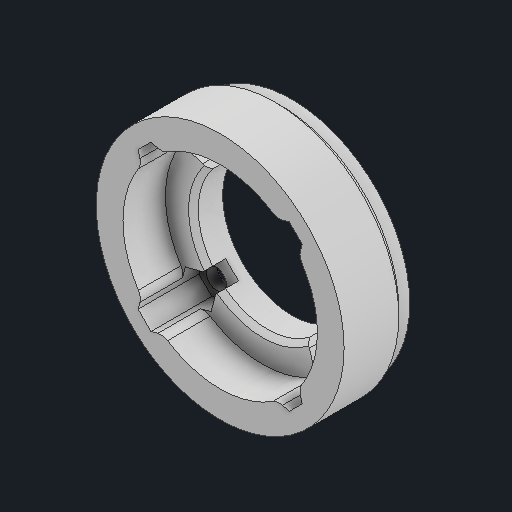
# Autodesk Inventor part: ShaftLock_A
Saved by Autodesk Inventor 2025.1 (Build 291241020, 241B)
## iProperties
Created: 2025-07-24
Part Number: ShaftLock_A
Material: 일반
Document SubType Name: Modeling
Designer: acalo
Density: 1 g/cm^3
Appearance: 기본값
Author: acalo
Autodesk Inventor part; units mm, degrees
ref_plane "YZ Plane" through (0, 0, 0) normal (1, 0, 0) x (0, 1, 0)
ref_plane "XZ Plane" through (0, 0, 0) normal (0, 1, 0) x (-1, 0, 0)
ref_plane "XY Plane" through (0, 0, 0) normal (0, 0, 1) x (1, 0, 0)
sketch "스케치1" plane through (0, 0, 0) normal (0, 0, 1) x (1, 0, 0)
  circle A0 centre (0, 0) radius 19.4
  circle A1 centre (10.6066, 10.6066) radius 1.65
  circle A2 centre (0, 0) radius 11
  circle A3 centre (-10.6066, 10.6066) radius 1.65
  circle A4 centre (-10.6066, -10.6066) radius 1.65
  circle A5 centre (10.6066, -10.6066) radius 1.65
  dimension "d1" = 22
  dimension "d5" = 360
  constraints: 6 centre point, 1 coincident, 9 other
  measures "d1" diameter of A2
extrude "돌출1" add sketch "스케치1" along normal blind 4.8
sketch "스케치2" plane through (0, 0, 4.8) normal (0, 0, 1) x (1, 0, 0)
  circle A0 centre (0, 0) radius 19.4 projected
  circle A1 centre (10.6066, -10.6066) radius 1.65 projected
  circle A2 centre (-10.6066, -10.6066) radius 1.65 projected
  circle A3 centre (-10.6066, 10.6066) radius 1.65 projected
  circle A4 centre (0, 0) radius 11 projected
  circle A5 centre (10.6066, 10.6066) radius 1.65 projected
  line L0 (10.6066, 10.6066) -> (8.8388, 8.8388)
  line L1 (10.6066, 10.6066) -> (13.1066, 10.6066) construction
  line L2 (7.8182, 9.8595) -> (8.5654, 12.6478)
  line L3 (8.5654, 12.6478) -> (11.3537, 13.395)
  line L4 (11.3537, 13.395) -> (13.395, 11.3537)
  line L5 (13.395, 11.3537) -> (12.6478, 8.5654)
  line L6 (12.6478, 8.5654) -> (9.8595, 7.8182)
  line L7 (9.8595, 7.8182) -> (7.8182, 9.8595)
  line L8 (-10.6066, 10.6066) -> (-10.6066, 13.1066) construction
  line L9 (-13.395, 11.3537) -> (-11.3537, 13.395)
  line L10 (-11.3537, 13.395) -> (-8.5654, 12.6478)
  line L11 (-8.5654, 12.6478) -> (-7.8182, 9.8595)
  line L12 (-7.8182, 9.8595) -> (-9.8595, 7.8182)
  line L13 (-12.6478, 8.5654) -> (-13.395, 11.3537)
  line L14 (-9.8595, 7.8182) -> (-12.6478, 8.5654)
  line L15 (-10.6066, -10.6066) -> (-13.1066, -10.6066) construction
  line L16 (-11.3537, -13.395) -> (-13.395, -11.3537)
  line L17 (-13.395, -11.3537) -> (-12.6478, -8.5654)
  line L18 (-12.6478, -8.5654) -> (-9.8595, -7.8182)
  line L19 (-9.8595, -7.8182) -> (-7.8182, -9.8595)
  line L20 (-8.5654, -12.6478) -> (-11.3537, -13.395)
  line L21 (-7.8182, -9.8595) -> (-8.5654, -12.6478)
  line L22 (10.6066, -10.6066) -> (10.6066, -13.1066) construction
  line L23 (13.395, -11.3537) -> (11.3537, -13.395)
  line L24 (11.3537, -13.395) -> (8.5654, -12.6478)
  line L25 (8.5654, -12.6478) -> (7.8182, -9.8595)
  line L26 (7.8182, -9.8595) -> (9.8595, -7.8182)
  line L27 (12.6478, -8.5654) -> (13.395, -11.3537)
  line L28 (9.8595, -7.8182) -> (12.6478, -8.5654)
  point P0 (-8.8388, 8.8388)
  point P1 (-8.8388, -8.8388)
  point P2 (8.8388, -8.8388)
  dimension "d9" = 2.5
  dimension "d10" = 135
  dimension "d13" = 360
  constraints: 58 end point, 1 coincident, 1 equal length, 1 horizontal, 1 midpoint, 78 other
  measures "d9" distance of L0.start L0.end
  measures "d10" angle of L0 L1
extrude "돌출2" cut sketch "스케치2" against normal blind 3 contours A1 | A2 | A3 | A5 | L7 L2 L3 L4 L5 L6 | L9 L10 L11 L12 L14 L13 | L16 L17 L18 L19 L21 L20 | L23 L24 L25 L26 L28 L27
sketch "스케치3" plane through (0, 0, 4.8) normal (0, 0, 1) x (1, 0, 0)
  circle A0 centre (0, 0) radius 16
  circle A1 centre (0, 0) radius 22.4
  line L0 (-7.8182, 9.8595) -> (-9.8595, 7.8182) projected
  line L1 (-9.8595, 7.8182) -> (-12.6478, 8.5654) projected
  line L2 (-12.6478, 8.5654) -> (-13.395, 11.3537) projected
  line L3 (-13.395, 11.3537) -> (-11.3537, 13.395) projected
  line L4 (-11.3537, 13.395) -> (-8.5654, 12.6478) projected
  line L5 (-8.5654, 12.6478) -> (-7.8182, 9.8595) projected
  line L6 (-9.8595, -7.8182) -> (-7.8182, -9.8595) projected
  line L7 (-7.8182, -9.8595) -> (-8.5654, -12.6478) projected
  line L8 (-8.5654, -12.6478) -> (-11.3537, -13.395) projected
  line L9 (-11.3537, -13.395) -> (-13.395, -11.3537) projected
  line L10 (-13.395, -11.3537) -> (-12.6478, -8.5654) projected
  line L11 (-12.6478, -8.5654) -> (-9.8595, -7.8182) projected
  line L12 (13.395, 11.3537) -> (12.6478, 8.5654) projected
  line L13 (12.6478, 8.5654) -> (9.8595, 7.8182) projected
  line L14 (9.8595, 7.8182) -> (7.8182, 9.8595) projected
  line L15 (7.8182, 9.8595) -> (8.5654, 12.6478) projected
  line L16 (8.5654, 12.6478) -> (11.3537, 13.395) projected
  line L17 (11.3537, 13.395) -> (13.395, 11.3537) projected
  line L18 (7.8182, -9.8595) -> (9.8595, -7.8182) projected
  line L19 (9.8595, -7.8182) -> (12.6478, -8.5654) projected
  line L20 (12.6478, -8.5654) -> (13.395, -11.3537) projected
  line L21 (13.395, -11.3537) -> (11.3537, -13.395) projected
  line L22 (11.3537, -13.395) -> (8.5654, -12.6478) projected
  line L23 (8.5654, -12.6478) -> (7.8182, -9.8595) projected
  circle A2 centre (0, 0) radius 19.4 projected
  circle A3 centre (0, 0) radius 11 projected
  point P0 (-9.4762, 12.8919)
  point P1 (9.4762, 12.8919)
  point P2 (12.8919, 9.4762)
  point P3 (12.8919, -9.4762)
  point P4 (9.4762, -12.8919)
  point P5 (-9.4762, -12.8919)
  point P6 (-12.8919, -9.4762)
  point P7 (-12.8919, 9.4762)
  dimension "d17" = 32
  dimension "d18" = 6.4
  constraints: 2 centre point, 1 coincident
  measures "d17" diameter of A0
  measures "d18" radial gap between concentric circles of A0 A1
extrude "돌출3" add sketch "스케치3" along normal blind 7 contours A1 | A2
chamfer "모따기1" distance 3 angle 45 1 edges at (-19.4, 0, 4.8)
sketch "스케치4" plane through (0, 0, 4.8) normal (0, 0, 1) x (1, 0, 0)
  circle A0 centre (0, 0) radius 11 projected
  arc A1 (12.8919, -9.4762) -> (12.8919, 9.4762) centre (0, 0) ccw projected
  line L0 (12.8919, 9.4762) -> (12.6478, 8.5654) projected
  line L1 (12.6478, 8.5654) -> (9.8595, 7.8182) projected
  line L2 (9.8595, 7.8182) -> (7.8182, 9.8595) projected
  line L3 (7.8182, 9.8595) -> (8.5654, 12.6478) projected
  line L4 (8.5654, 12.6478) -> (9.4762, 12.8919) projected
  arc A2 (9.4762, 12.8919) -> (-9.4762, 12.8919) centre (0, 0) ccw projected
  line L5 (-9.4762, 12.8919) -> (-8.5654, 12.6478) projected
  line L6 (-8.5654, 12.6478) -> (-7.8182, 9.8595) projected
  line L7 (-7.8182, 9.8595) -> (-9.8595, 7.8182) projected
  line L8 (-9.8595, 7.8182) -> (-12.6478, 8.5654) projected
  line L9 (-12.6478, 8.5654) -> (-12.8919, 9.4762) projected
  arc A3 (-12.8919, 9.4762) -> (-12.8919, -9.4762) centre (0, 0) ccw projected
  line L10 (-12.8919, -9.4762) -> (-12.6478, -8.5654) projected
  line L11 (-12.6478, -8.5654) -> (-9.8595, -7.8182) projected
  line L12 (-9.8595, -7.8182) -> (-7.8182, -9.8595) projected
  line L13 (-7.8182, -9.8595) -> (-8.5654, -12.6478) projected
  line L14 (-8.5654, -12.6478) -> (-9.4762, -12.8919) projected
  arc A4 (-9.4762, -12.8919) -> (9.4762, -12.8919) centre (0, 0) ccw projected
  line L15 (9.4762, -12.8919) -> (8.5654, -12.6478) projected
  line L16 (8.5654, -12.6478) -> (7.8182, -9.8595) projected
  line L17 (7.8182, -9.8595) -> (9.8595, -7.8182) projected
  line L18 (9.8595, -7.8182) -> (12.6478, -8.5654) projected
  line L19 (12.6478, -8.5654) -> (12.8919, -9.4762) projected
  circle A5 centre (0, 0) radius 11.4
  line L20 (9.8595, 7.8182) -> (9.0168, 6.9755)
  line L21 (8.8388, 8.8388) -> (8.4116, 8.4116)
  line L22 (7.8182, 9.8595) -> (6.9755, 9.0168)
  line L23 (-7.8182, 9.8595) -> (-6.9755, 9.0168)
  line L24 (-9.8595, 7.8182) -> (-9.0168, 6.9755)
  line L25 (-9.8595, -7.8182) -> (-9.0168, -6.9755)
  line L26 (-7.8182, -9.8595) -> (-6.9755, -9.0168)
  line L27 (7.8182, -9.8595) -> (6.9755, -9.0168)
  line L28 (9.8595, -7.8182) -> (9.0168, -6.9755)
  dimension "d24" = 0.4
  dimension "d27" = 360
  constraints: 18 end point, 1 midpoint, 1 parallel, 1 perpendicular, 1 symmetric about line, 28 other
extrude "돌출4" cut sketch "스케치4" against normal blind 7 contours A5
extrude "돌출5" cut sketch "스케치4" against normal up to surface (3 mm away) contours L17 L27 A5 L28 | L20 A5 L22 L2 | L26 L12 L25 A5 | A5 L24 L7 L23
sketch "스케치5" plane through (0, 0, 11.8) normal (0, 0, 1) x (1, 0, 0)
  circle A0 centre (0, 0) radius 22.4 projected
  circle A1 centre (0, 0) radius 20.4
  dimension "d33" = 2
  constraints: 1 centre point
  measures "d33" radial gap between concentric circles of A0 A1
extrude "돌출6" cut sketch "스케치5" against normal blind 10
sketch "스케치6" plane through (0, 0, 4.8) normal (0, 0, 1) x (1, 0, 0)
  circle A0 centre (0, 0) radius 12.2
  dimension "d36" = 24.4
  constraints: 1 centre point, 1 coincident
  measures "d36" diameter of A0
extrude "돌출7" cut sketch "스케치6" against normal blind 0.8
chamfer "모따기2" distance 0.8 angle 45 4 edges at (12.2, 0, 4) (0, -12.2, 4) (0, 12.2, 4) (-12.2, 0, 4)
sketch "스케치7" plane through (0, 0, 11.8) normal (0, 0, 1) x (1, 0, 0)
  circle A0 centre (0, 0) radius 20.4 projected
  line L0 (-13.395, 11.3537) -> (-11.3537, 13.395) projected
  line L1 (-11.3537, 13.395) -> (-9.4762, 12.8919) projected
  arc A1 (9.4762, 12.8919) -> (-9.4762, 12.8919) centre (0, 0) ccw projected
  line L2 (9.4762, 12.8919) -> (11.3537, 13.395) projected
  line L3 (11.3537, 13.395) -> (13.395, 11.3537) projected
  line L4 (13.395, 11.3537) -> (12.8919, 9.4762) projected
  arc A2 (12.8919, -9.4762) -> (12.8919, 9.4762) centre (0, 0) ccw projected
  line L5 (12.8919, -9.4762) -> (13.395, -11.3537) projected
  line L6 (13.395, -11.3537) -> (11.3537, -13.395) projected
  line L7 (11.3537, -13.395) -> (9.4762, -12.8919) projected
  arc A3 (-9.4762, -12.8919) -> (9.4762, -12.8919) centre (0, 0) ccw projected
  line L8 (-9.4762, -12.8919) -> (-11.3537, -13.395) projected
  line L9 (-11.3537, -13.395) -> (-13.395, -11.3537) projected
  line L10 (-13.395, -11.3537) -> (-12.8919, -9.4762) projected
  arc A4 (-12.8919, 9.4762) -> (-12.8919, -9.4762) centre (0, 0) ccw projected
  line L11 (-12.8919, 9.4762) -> (-13.395, 11.3537) projected
  circle A5 centre (10.6066, 10.6066) radius 1.65 projected
  line L12 (10.6066, 10.6066) -> (13.118, 9.9337)
  line L13 (12.7295, 8.4837) -> (9.8296, 7.7067)
  line L14 (7.7067, 9.8296) -> (8.4837, 12.7295)
  line L15 (8.4837, 12.7295) -> (11.3836, 13.5065)
  line L16 (11.3836, 13.5065) -> (13.5065, 11.3836)
  line L17 (13.5065, 11.3836) -> (12.7295, 8.4837)
  line L18 (7.7067, 9.8296) -> (6.6452, 8.7681)
  line L19 (6.6452, 8.7681) -> (8.7681, 6.6452)
  line L20 (8.7681, 6.6452) -> (9.8296, 7.7067)
  point P0 (9.3724, 12.9676)
  point P1 (12.9676, 9.3724)
  dimension "d42" = 2.6
  constraints: 18 end point, 3 perpendicular, 1 coincident, 1 midpoint, 11 other
  measures "d42" distance of L12.start L12.end
extrude "돌출8" cut sketch "스케치7" against normal up to surface (10 mm away) contours L15 L16 L17 L12 L4 L3 L2 A1 | A1 L2 L3 L4 A2 L17 L13 L20 L19 L18 L14 L15 | L17 A2 L4 L12
pattern_circular "원형 패턴1" count 4 over 360 about axis through (0, 0, 4.8) along (0, 0, -1) of "돌출8"
fillet "모깎기1" radius 2 8 edges at (12.9676, 9.3724, 8.3) (9.3724, 12.9676, 8.3) (12.9676, -9.3724, 8.3) (9.3724, -12.9676, 8.3) (-9.3724, -12.9676, 8.3) (-12.9676, -9.3724, 8.3) (-12.9676, 9.3724, 8.3) (-9.3724, 12.9676, 8.3)
